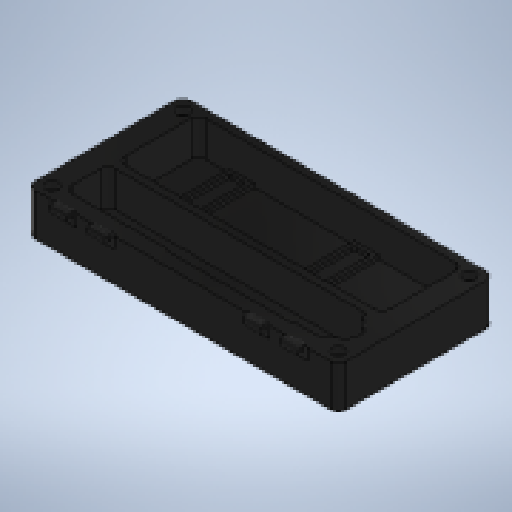
# Autodesk Inventor part: PinecilCaseBottom
Saved by Autodesk Inventor 2026 (Build 300175050, 175E)
## iProperties
Created: 2025-10-09
Part Number: PinecilCaseBottom
Material: Generic
Document SubType Name: Modeling
Designer: Nicholas M
Density: 1 g/cm^3
Appearance: Smooth - Black
Author: Nicholas M
Autodesk Inventor part; units mm, degrees
ref_plane "YZ Plane" through (0, 0, 0) normal (1, 0, 0) x (0, 1, 0)
sketch "Sketch1" plane through (0, 0, 0) normal (0, 1, 0) x (-1, 0, 0)
  line L0 (0, 0) -> (127, 0)
  line L1 (127, 0) -> (127, -63.5)
  line L2 (127, -63.5) -> (0, -63.5)
  line L3 (0, -63.5) -> (0, 0)
  line L4 (123.825, -60.325) -> (123.825, -3.175)
  line L5 (123.825, -3.175) -> (3.175, -3.175)
  line L6 (3.175, -3.175) -> (3.175, -60.325)
  line L7 (3.175, -60.325) -> (123.825, -60.325)
  dimension "d0" = 127
  dimension "d1" = 63.5
  dimension "d2" = 3.175
  constraints: 16 end point, 4 parallel, 2 perpendicular, 1 horizontal, 3 other
  measures "d0" distance of L1.end L2.end
  measures "d1" distance of L2.end L0.start
  measures "d2" distance between parallel lines of L1 L4
extrude "Extrusion1" add sketch "Sketch1" along normal blind 3.175 contours L0 L1 L2 L3 | L7 L6 L5 L4
extrude "Extrusion2" add sketch "Sketch1" along normal blind 17.78
fillet "Fillet1" radius 3.175 8 edges at (0, 8.89, 0) (0, 8.89, -63.5) (-127, 8.89, -63.5) (-127, 8.89, 0) (-123.825, 10.4775, -3.175) (-3.175, 10.4775, -3.175) (-123.825, 10.4775, -60.325) (-3.175, 10.4775, -60.325)
sketch "Sketch2" plane through (0, 3.175, 0) normal (0, 1, 0) x (1, 0, 0)
  line L0 (-120.65, 6.35) -> (-12.7, 6.35)
  line L1 (-12.7, 6.35) -> (-12.7, 24.13)
  line L2 (-12.7, 24.13) -> (-120.65, 24.13)
  line L3 (-120.65, 24.13) -> (-120.65, 6.35)
  line L4 (-3.175, 57.15) -> (-3.175, 6.35) projected
  line L5 (-6.35, 3.175) -> (-120.65, 3.175) projected
  line L6 (-24.892, 6.35) -> (-75.692, 6.35)
  line L7 (-75.692, 6.35) -> (-75.692, 5.588) construction
  line L8 (-75.692, 5.588) -> (-24.892, 5.588)
  line L9 (-24.892, 5.588) -> (-24.892, 6.35) construction
  line L10 (-24.892, 5.588) -> (-24.13, 6.35)
  line L11 (-123.825, 6.35) -> (-123.825, 57.15) projected
  line L12 (-75.692, 5.588) -> (-76.454, 6.35)
  line L13 (-123.825, 27.305) -> (-3.175, 27.305)
  arc A0 (-3.175, 57.15) -> (-6.35, 60.325) centre (-6.35, 57.15) ccw projected
  line L14 (-6.35, 60.325) -> (-120.65, 60.325) projected
  arc A1 (-120.65, 60.325) -> (-123.825, 57.15) centre (-120.65, 57.15) ccw projected
  line L15 (-123.825, 57.15) -> (-123.825, 6.35) projected
  arc A2 (-123.825, 6.35) -> (-120.65, 3.175) centre (-120.65, 6.35) ccw projected
  line L16 (-120.65, 3.175) -> (-6.35, 3.175) projected
  arc A3 (-6.35, 3.175) -> (-3.175, 6.35) centre (-6.35, 6.35) ccw projected
  line L17 (-3.175, 6.35) -> (-3.175, 57.15) projected
  point P0 (0, 0)
  dimension "d8" = 107.95
  dimension "d9" = 17.78
  dimension "d11" = 3.175
  dimension "d13" = 18.542
  dimension "d14" = 11.43
  dimension "d15" = 3.175
  dimension "d16" = 45
  dimension "d17" = 50.8
  dimension "d18" = 45
  dimension "d20" = 3.175
  constraints: 22 end point, 5 parallel, 5 point on line, 2 horizontal, 2 perpendicular
  measures "d8" distance of L2.end L1.end
  measures "d9" distance of L1.end L0.end
  measures "d11" distance between parallel lines of L5 L0
  measures "d13" distance between parallel lines of L2 L8
  measures "d14" distance of L0.end L10.end
  measures "d15" distance between parallel lines of L11 L3
  measures "d16" angle of L9 L10
  measures "d17" distance of L7.end L8.end
  measures "d18" angle of L7 L12
  measures "d20" distance between parallel lines of L2 L13
extrude "Extrusion3" add sketch "Sketch2" along normal blind 11.684 contours L4 A3 L5 A2 L11 L13
chamfer "Chamfer1" distance 5.08 angle 45 1 edges at (-120.65, 9.017, -6.35)
fillet "Fillet2" radius 0.7937 9 edges at (-76.454, 9.017, -6.35) (-75.692, 9.017, -5.588) (-24.892, 9.017, -5.588) (-24.13, 9.017, -6.35) (-12.7, 9.017, -6.35) (-12.7, 9.017, -24.13) (-120.65, 9.017, -24.13) (-120.65, 9.017, -11.43) (-115.57, 9.017, -6.35)
sketch "Sketch3" plane through (0, 14.859, 0) normal (0, 1, 0) x (1, 0, 0)
  line L0 (-12.7, 23.3363) -> (-12.7, 7.1438) projected
  circle A0 centre (-12.7, 15.24) radius 6.35
  line L1 (-3.175, 27.305) -> (-3.175, 6.35) projected
  line L2 (-3.175, 27.305) -> (-123.825, 27.305) projected
  line L3 (-123.825, 6.35) -> (-123.825, 27.305) projected
  arc A1 (-23.8012, 6.35) -> (-24.3625, 6.1175) centre (-23.8012, 5.5563) ccw projected
  line L4 (-24.3625, 6.1175) -> (-24.6595, 5.8205) projected
  arc A2 (-25.2208, 5.588) -> (-24.6595, 5.8205) centre (-25.2208, 6.3818) ccw projected
  line L5 (-25.2208, 5.588) -> (-75.3632, 5.588) projected
  arc A3 (-75.9245, 5.8205) -> (-75.3632, 5.588) centre (-75.3632, 6.3818) ccw projected
  line L6 (-75.9245, 5.8205) -> (-76.2215, 6.1175) projected
  arc A4 (-76.2215, 6.1175) -> (-76.7828, 6.35) centre (-76.7828, 5.5563) ccw projected
  line L7 (-76.7828, 6.35) -> (-115.2412, 6.35) projected
  arc A5 (-115.8025, 6.5825) -> (-115.2412, 6.35) centre (-115.2412, 7.1438) ccw projected
  line L8 (-120.4175, 11.1975) -> (-115.8025, 6.5825) projected
  arc A6 (-120.65, 11.7588) -> (-120.4175, 11.1975) centre (-119.8562, 11.7588) ccw projected
  line L9 (-120.65, 11.7588) -> (-120.65, 23.3363) projected
  arc A7 (-119.8562, 24.13) -> (-120.65, 23.3363) centre (-119.8562, 23.3363) ccw projected
  line L10 (-119.8562, 24.13) -> (-13.4937, 24.13) projected
  arc A8 (-12.7, 23.3363) -> (-13.4937, 24.13) centre (-13.4937, 23.3363) ccw projected
  line L11 (-12.7, 23.3363) -> (-12.7, 7.1438) projected
  arc A9 (-13.4937, 6.35) -> (-12.7, 7.1438) centre (-13.4937, 7.1438) ccw projected
  line L12 (-13.4937, 6.35) -> (-23.8012, 6.35) projected
  line L13 (-6.35, 5.5563) -> (-6.35, 25.4813)
  line L14 (-6.35, 3.175) -> (-120.65, 3.175) projected
  arc A10 (-6.35, 3.175) -> (-3.175, 6.35) centre (-6.35, 6.35) ccw projected
  arc A11 (-123.825, 6.35) -> (-120.65, 3.175) centre (-120.65, 6.35) ccw projected
  point P0 (0, 0)
  point P1 (-12.7, 21.59)
  point P2 (-12.7, 8.89)
  dimension "d27" = 3.175
  constraints: 2 end point, 1 centre point, 1 midpoint, 1 tangent, 1 vertical
  measures "d27" distance between parallel lines of L1 L13
revolve "Revolution1" cut sketch "Sketch3" angle 360 about axis through (-12.7, 14.859, -23.3363) along (0, 0, 1) picked at (-11.7816, 17.1471) contours A0 L0
fillet "Fillet3" radius 0.7937 1 edges at (-12.7, 8.509, -15.24)
sketch "Sketch4" plane through (0, 3.175, 0) normal (0, 1, 0) x (1, 0, 0)
  line L0 (-102.87, 29.21) -> (-96.52, 29.21)
  line L1 (-96.52, 29.21) -> (-96.52, 58.42)
  line L2 (-96.52, 58.42) -> (-102.87, 58.42)
  line L3 (-102.87, 58.42) -> (-102.87, 29.21)
  line L4 (-52.07, 29.21) -> (-45.72, 29.21)
  line L5 (-45.72, 29.21) -> (-45.72, 58.42)
  line L6 (-45.72, 58.42) -> (-52.07, 58.42)
  line L7 (-52.07, 58.42) -> (-52.07, 29.21)
  line L8 (-120.65, 60.325) -> (-6.35, 60.325) projected
  line L9 (-123.825, 6.35) -> (-123.825, 57.15) projected
  line L10 (-123.825, 27.305) -> (-3.175, 27.305) projected
  line L11 (-3.175, 27.305) -> (-3.175, 57.15) projected
  arc A0 (-3.175, 57.15) -> (-6.35, 60.325) centre (-6.35, 57.15) ccw projected
  line L12 (-6.35, 60.325) -> (-120.65, 60.325) projected
  arc A1 (-120.65, 60.325) -> (-123.825, 57.15) centre (-120.65, 57.15) ccw projected
  line L13 (-123.825, 57.15) -> (-123.825, 27.305) projected
  line L14 (-96.393, 58.547) -> (-96.393, 29.083)
  line L15 (-96.393, 29.083) -> (-102.997, 29.083)
  line L16 (-102.997, 29.083) -> (-102.997, 58.547)
  line L17 (-102.997, 58.547) -> (-96.393, 58.547)
  line L18 (-52.197, 29.083) -> (-45.593, 29.083)
  line L19 (-45.593, 29.083) -> (-45.593, 58.547)
  line L20 (-45.593, 58.547) -> (-52.197, 58.547)
  line L21 (-52.197, 58.547) -> (-52.197, 29.083)
  line L22 (-43.815, 60.325) -> (-43.815, 27.305)
  line L23 (-43.815, 27.305) -> (-53.975, 27.305)
  line L24 (-53.975, 27.305) -> (-53.975, 60.325)
  line L25 (-53.975, 60.325) -> (-43.815, 60.325)
  line L26 (-94.615, 60.325) -> (-94.615, 27.305)
  line L27 (-94.615, 27.305) -> (-104.775, 27.305)
  line L28 (-104.775, 27.305) -> (-104.775, 60.325)
  line L29 (-104.775, 60.325) -> (-94.615, 60.325)
  line L30 (-3.175, 27.305) -> (-123.825, 27.305) projected
  point P0 (0, 0)
  point P1 (-99.695, 58.42)
  point P2 (-48.895, 58.42)
  dimension "d30" = 6.35
  dimension "d32" = 6.35
  dimension "d34" = 50.8
  dimension "d35" = 1.905
  dimension "d40" = 0.127
  dimension "d41" = 0.127
  dimension "d42" = 1.905
  dimension "d43" = 1.905
  dimension "d53" = 19.05
  constraints: 48 end point, 12 parallel, 6 perpendicular, 2 collinear, 2 horizontal, 2 midpoint, 1 horizontal alignment, 12 other
  measures "d30" distance of L2.end L1.end
  measures "d32" distance of L6.end L5.end
  measures "d34" distance of point (-99.695, 58.42) point (-48.895, 58.42)
  measures "d35" distance between parallel lines of L8 L6
  measures "d40" distance between parallel lines of L1 L14
  measures "d41" distance between parallel lines of L7 L21
  measures "d42" distance between parallel lines of L5 L22
  measures "d43" distance between parallel lines of L1 L26
  measures "d53" distance between parallel lines of L9 L28
extrude "Extrusion4" add sketch "Sketch4" along normal blind 1.5875 contours L8 L26 L10 L28 | L8 L22 L10 L24
fillet "Fillet4" radius 0.7937 8 edges at (-52.197, 3.9688, -29.083) (-45.593, 3.9688, -29.083) (-45.593, 3.9688, -58.547) (-52.197, 3.9688, -58.547) (-96.393, 3.9688, -58.547) (-102.997, 3.9688, -58.547) (-102.997, 3.9688, -29.083) (-96.393, 3.9688, -29.083)
ref_plane "Work Plane1" through (-12.7, 0, -3.175) normal (1, 0, 0) x (0, 0, -1)
sketch "Sketch5" plane through (-12.7, 0, -3.175) normal (1, 0, 0) x (0, 0, -1)
  line L0 (0, 17.78) -> (-3.175, 17.78) projected
  line L1 (-3.175, 17.78) -> (-3.175, 0) projected
  line L2 (-3.175, 0) -> (0, 0) projected
  line L3 (0, 0) -> (0, 17.78) projected
  line L4 (57.15, 17.78) -> (57.15, 0) projected
  line L5 (0, 17.78) -> (57.15, 17.78) projected
  line L6 (0, 0) -> (0, 17.78) projected
  line L7 (0, 0) -> (57.15, 0) projected
  circle A0 centre (-5.08, 17.78) radius 1.905
  line L8 (-3.175, 17.78) -> (-3.175, 0) projected
  circle A1 centre (-5.08, 17.78) radius 0.635
  line L9 (-6.427, 16.433) -> (-3.175, 13.1809)
  dimension "d45" = 3.81
  dimension "d46" = 1.27
  dimension "d47" = 45
  constraints: 2 end point, 1 centre point, 1 coincident, 1 horizontal alignment, 1 point on line, 1 vertical, 4 other
  measures "d46" diameter of A1
  measures "d47" angle of L1 L9
extrude "Extrusion5" add sketch "Sketch5" against normal blind 7.493 contours A0 | L1 L9 A0
ref_plane "Work Plane2" through (-35.56, 0, -3.175) normal (1, 0, 0) x (0, 0, -1)
extrude "Extrusion6" add sketch "Sketch5" along normal blind 7.493 from surface at -22.86 contours A0 | L1 L9 A0
ref_plane "Work Plane3" through (-63.5, 0, -3.175) normal (1, 0, 0) x (0, 0, -1)
mirror "Mirror1" about plane through (-63.5, 0, -3.175) normal (1, 0, 0) of "Extrusion5", "Extrusion6"
sketch "Sketch6" plane through (0, 3.175, 0) normal (0, 1, 0) x (1, 0, 0)
  line L0 (-43.815, 27.305) -> (-3.175, 27.305) projected
  line L1 (-24.765, 27.305) -> (-24.765, 60.325)
  line L2 (-43.815, 27.305) -> (-43.815, 60.325) projected
  line L3 (-21.59, 27.305) -> (-21.59, 60.325)
  line L4 (-120.65, 60.325) -> (-6.35, 60.325) projected
  line L5 (-123.825, 57.15) -> (-123.825, 27.305) projected
  line L6 (-123.825, 27.305) -> (-117.475, 27.305)
  line L7 (-117.475, 27.305) -> (-117.475, 60.325)
  line L8 (-117.475, 60.325) -> (-123.825, 60.325)
  line L9 (-123.825, 60.325) -> (-123.825, 27.305)
  line L10 (-3.175, 57.15) -> (-3.175, 27.305) projected
  line L11 (-3.175, 27.305) -> (-9.525, 27.305)
  line L12 (-9.525, 27.305) -> (-9.525, 60.325)
  line L13 (-9.525, 60.325) -> (-3.175, 60.325)
  line L14 (-3.175, 60.325) -> (-3.175, 27.305)
  point P0 (0, 0)
  dimension "d54" = 19.05
  dimension "d55" = 3.175
  dimension "d80" = 6.35
  dimension "d81" = 6.35
  constraints: 20 end point, 6 point on line, 5 parallel, 2 horizontal, 2 perpendicular, 1 collinear, 1 vertical
  measures "d54" distance between parallel lines of L2 L1
  measures "d55" distance between parallel lines of L1 L3
  measures "d80" distance of L5.end L6.end
  measures "d81" distance of L12.end L13.end
extrude "Extrusion7" add sketch "Sketch6" along normal up to surface (14.605 mm away) contours L12 L4 L13 L14 L10 L0 | L4 L7 L6 L5 L9 L8
fillet "Fillet5" radius 3.175 4 edges at (-117.475, 9.017, -27.305) (-117.475, 10.4775, -60.325) (-9.525, 9.017, -27.305) (-9.525, 10.4775, -60.325)
fillet "Fillet6" radius 0.7937 8 edges at (-0.9299, 0, -62.5701) (-63.5, 0, -63.5) (-126.0701, 0, -62.5701) (-127, 0, -31.75) (-126.0701, 0, -0.9299) (-63.5, 0, 0) (-0.9299, 0, -0.9299) (0, 0, -31.75)
sketch "Sketch10" plane through (0, 17.78, 0) normal (0, 1, 0) x (1, 0, 0)
  circle A0 centre (-5.08, 5.08) radius 2.54
  line L0 (0, 3.175) -> (0, 60.325) projected
  line L1 (-12.7, 0) -> (-3.175, 0) projected
  circle A1 centre (-121.92, 5.08) radius 2.54
  line L2 (-127, 60.325) -> (-127, 3.175) projected
  line L3 (-123.825, 0) -> (-114.3, 0) projected
  circle A2 centre (-5.08, 58.42) radius 2.54
  line L4 (-3.175, 63.5) -> (-123.825, 63.5) projected
  circle A3 centre (-121.92, 58.42) radius 2.54
  point P0 (0, 0)
  dimension "d74" = 5.08
  dimension "d75" = 5.08
  dimension "d76" = 5.08
  dimension "d77" = 5.08
  dimension "d78" = 5.08
  dimension "d79" = 5.08
  dimension "d82" = 5.08
  dimension "d83" = 5.08
  dimension "d84" = 5.08
  dimension "d85" = 5.08
  dimension "d86" = 5.08
  dimension "d87" = 5.08
  constraints: 4 centre point
  measures "d74" diameter of A0
  measures "d75" distance from line of L0 A0.centre
  measures "d76" distance from line of L1 A0.centre
  measures "d77" diameter of A1
  measures "d78" distance from line of L2 A1.centre
  measures "d79" distance from line of L3 A1.centre
  measures "d82" diameter of A2
  measures "d83" distance from line of L4 A2.centre
  measures "d84" distance from line of L0 A2.centre
  measures "d85" diameter of A3
  measures "d86" distance from line of L4 A3.centre
  measures "d87" distance from line of L2 A3.centre
extrude "Extrusion11" cut sketch "Sketch10" against normal blind 3
sketch "Sketch11" plane through (0, 14.859, 0) normal (0, 1, 0) x (1, 0, 0)
  arc A0 (-3.175, 6.7601) -> (-6.7601, 3.175) centre (-5.08, 5.08) ccw projected
  line L0 (-3.175, 27.305) -> (-3.175, 6.7601) projected
  line L1 (-3.175, 27.305) -> (-9.525, 27.305) projected
  line L2 (-9.525, 30.48) -> (-9.525, 27.305) projected
  arc A1 (-12.7, 27.305) -> (-9.525, 30.48) centre (-12.7, 30.48) ccw projected
  line L3 (-12.7, 27.305) -> (-114.3, 27.305) projected
  arc A2 (-117.475, 30.48) -> (-114.3, 27.305) centre (-114.3, 30.48) ccw projected
  line L4 (-117.475, 27.305) -> (-117.475, 30.48) projected
  line L5 (-117.475, 27.305) -> (-123.825, 27.305) projected
  line L6 (-123.825, 6.7601) -> (-123.825, 27.305) projected
  arc A3 (-120.2399, 3.175) -> (-123.825, 6.7601) centre (-121.92, 5.08) ccw projected
  line L7 (-6.7601, 3.175) -> (-120.2399, 3.175) projected
  line L8 (-25.2208, 5.588) -> (-75.3632, 5.588) projected
  arc A4 (-75.9245, 5.8205) -> (-75.3632, 5.588) centre (-75.3632, 6.3818) ccw projected
  line L9 (-75.9245, 5.8205) -> (-76.2215, 6.1175) projected
  arc A5 (-76.2215, 6.1175) -> (-76.7828, 6.35) centre (-76.7828, 5.5563) ccw projected
  line L10 (-76.7828, 6.35) -> (-115.2412, 6.35) projected
  arc A6 (-115.8025, 6.5825) -> (-115.2412, 6.35) centre (-115.2412, 7.1438) ccw projected
  line L11 (-120.4175, 11.1975) -> (-115.8025, 6.5825) projected
  arc A7 (-120.65, 11.7588) -> (-120.4175, 11.1975) centre (-119.8562, 11.7588) ccw projected
  line L12 (-120.65, 11.7588) -> (-120.65, 23.3363) projected
  arc A8 (-119.8562, 24.13) -> (-120.65, 23.3363) centre (-119.8562, 23.3363) ccw projected
  line L13 (-119.8562, 24.13) -> (-13.4937, 24.13) projected
  arc A9 (-12.7, 23.3363) -> (-13.4937, 24.13) centre (-13.4937, 23.3363) ccw projected
  line L14 (-12.7, 23.3363) -> (-12.7, 22.3395) projected
  arc A10 (-12.7, 22.3395) -> (-11.9944, 21.5507) centre (-11.9062, 22.3395) ccw projected
  arc A11 (-11.9944, 8.9293) -> (-11.9944, 21.5507) centre (-12.7, 15.24) ccw projected
  arc A12 (-11.9944, 8.9293) -> (-12.7, 8.1405) centre (-11.9062, 8.1405) ccw projected
  line L15 (-12.7, 8.1405) -> (-12.7, 7.1438) projected
  arc A13 (-13.4937, 6.35) -> (-12.7, 7.1438) centre (-13.4937, 7.1438) ccw projected
  line L16 (-13.4937, 6.35) -> (-23.8012, 6.35) projected
  arc A14 (-23.8012, 6.35) -> (-24.3625, 6.1175) centre (-23.8012, 5.5563) ccw projected
  line L17 (-24.3625, 6.1175) -> (-24.6595, 5.8205) projected
  arc A15 (-25.2208, 5.588) -> (-24.6595, 5.8205) centre (-25.2208, 6.3818) ccw projected
  point P0 (0, 0)
extrude "Extrusion12" add sketch "Sketch11" along normal up to surface (2.921 mm away)
sketch "Sketch12" plane through (0, 17.78, 0) normal (0, 1, 0) x (1, 0, 0)
  line L0 (-120.65, 7.8991) -> (-118.11, 7.8991)
  line L1 (-118.11, 7.8991) -> (-118.11, 24.7663)
  line L2 (-118.11, 24.7663) -> (-120.65, 24.7663)
  line L3 (-120.65, 24.7663) -> (-120.65, 7.8991)
  line L4 (-120.65, 23.3363) -> (-120.65, 11.7588)
  point P0 (0, 0)
  dimension "d92" = 2.54
  constraints: 10 end point, 2 parallel, 1 collinear, 1 horizontal, 1 perpendicular
  measures "d92" distance of L2.end L1.end
extrude "Extrusion13" add sketch "Sketch12" against normal up to surface (14.605 mm away)
fillet "Fillet9" radius 3.175 2 edges at (-118.11, 16.3195, -24.13) (-118.11, 9.017, -24.13)
fillet "Fillet10" radius 0.7937 2 edges at (-118.11, 16.3195, -8.89) (-118.11, 9.017, -8.89)
body "Solid1"
